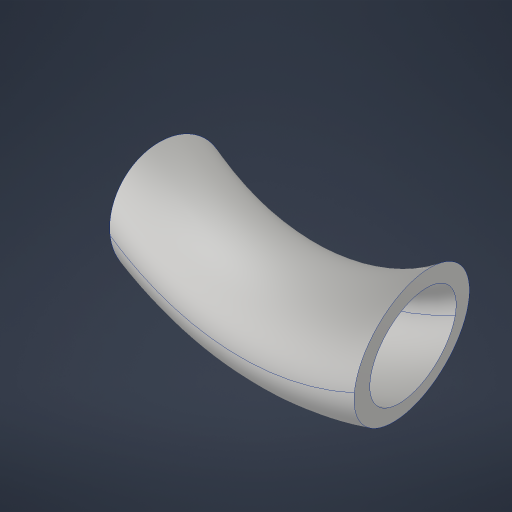
# Autodesk Inventor part: EL2-024
Saved by Autodesk Inventor 2023.4 (Build 274418000, 418)
## iProperties
Created: 2025-02-10
Part Number: EL2-024
Material: Aluminum 6061
Document SubType Name: Modeling
Designer: brand
Density: 2.7 g/cm^3
Appearance: Aluminum - Flat
Author: brand
Autodesk Inventor part; units mm, degrees
ref_plane "YZ Plane" through (0, 0, 0) normal (1, 0, 0) x (0, 1, 0)
ref_plane "XZ Plane" through (0, 0, 0) normal (0, 1, 0) x (-1, 0, 0)
ref_plane "XY Plane" through (0, 0, 0) normal (0, 0, 1) x (1, 0, 0)
sketch "Sketch1" plane through (0, 0, 0) normal (0, 0, 1) x (1, 0, 0)
  line L0 (-50.8, -41.275) -> (50.8, -41.275)
  line L1 (50.8, -41.275) -> (50.8, 41.275)
  line L2 (50.8, 41.275) -> (-50.8, 41.275)
  line L3 (-50.8, 41.275) -> (-50.8, -41.275)
  line L4 (-50.8, -41.275) -> (50.8, 41.275) construction
  line L5 (50.8, -41.275) -> (-50.8, 41.275) construction
  point P0 (0, 0)
  dimension "d0" = 101.6
  dimension "d1" = 82.55
  constraints: 12 end point, 2 midpoint, 2 parallel, 1 horizontal, 1 perpendicular
  measures "d0" distance of L2.end L1.end
  measures "d1" distance of L1.end L0.end
extrude "Extrusion1" add sketch "Sketch1" along normal mid plane 50.8
sketch "Sketch2" plane through (50.8, -41.275, 25.4) normal (1, 0, 0) x (0, 0, -1)
  line L0 (50.8, 82.55) -> (50.8, 0) construction
  line L1 (50.8, 0) -> (0, 0) construction
  line L2 (0, 0) -> (0, 82.55) construction
  line L3 (0, 82.55) -> (50.8, 82.55) construction
  circle A0 centre (25.4, 41.275) radius 19.05
  line L4 (50.8, 82.55) -> (0, 82.55) construction
  dimension "d4" = 38.1
  constraints: 3 coincident, 1 centre point
  measures "d4" diameter of A0
sketch "Sketch3" plane through (0, 0, 0) normal (0, 0, 1) x (1, 0, 0)
  line L0 (50.8, -41.275) -> (-50.8, -41.275) construction
  line L1 (-50.8, -41.275) -> (-50.8, 41.275) construction
  line L2 (-50.8, 41.275) -> (50.8, 41.275) construction
  line L3 (50.8, 41.275) -> (50.8, -41.275) construction
  arc A0 (-50.8, 0) -> (50.8, 0) centre (0, 80.5725) ccw construction
  circle A1 centre (0, 80.5725) radius 95.25
  point P0 (0, 0)
  dimension "d5" = 95.25
  constraints: 2 centre point, 2 point on circle, 1 coincident, 1 concentric, 1 horizontal alignment, 1 midpoint
  measures "d5" radius of A0
sweep "Sweep1" cut profiles "Sketch2" path "Sketch3"
sketch "Sketch7" plane through (50.8, -41.275, 25.4) normal (1, 0, 0) x (0, 0, -1)
  circle A0 centre (25.4, 41.275) radius 19.05 construction
  line L0 (50.8, 82.55) -> (50.8, 0) construction
  line L1 (50.8, 0) -> (0, 0) construction
  line L2 (0, 0) -> (0, 82.55) construction
  line L3 (0, 82.55) -> (50.8, 82.55) construction
  circle A1 centre (25.4, 41.275) radius 25.4
  line L4 (0, 0) -> (0, 82.55) construction
  line L5 (0, 41.275) -> (50.8, 41.275)
  line L6 (50.8, 41.275) -> (50.8, 107.95)
  line L7 (50.8, 107.95) -> (0, 107.95)
  line L8 (0, 107.95) -> (0, 41.275)
  line L9 (50.8, 82.55) -> (50.8, 0) construction
  line L10 (0, 41.275) -> (50.8, 41.275)
  line L11 (50.8, 41.275) -> (50.8, -25.4)
  line L12 (50.8, -25.4) -> (0, -25.4)
  line L13 (0, -25.4) -> (0, 41.275)
  point P0 (25.4, 41.275)
  point P1 (25.4, -25.4)
  dimension "d20" = 6.35
  dimension "d21" = 25.4
  dimension "d22" = 25.4
  constraints: 16 end point, 4 midpoint, 4 parallel, 2 horizontal, 2 perpendicular, 2 point on circle, 1 centre point, 1 coincident
  measures "d20" radial gap between concentric circles of A1 A0
  measures "d21" distance between parallel lines of L7 L3
  measures "d22" distance from line of point (25.4, -25.4) L1
sweep "Sweep5" cut profiles "Sketch7" path "Sketch3" contours A1 L8 L7 L6
sweep "Sweep6" cut profiles "Sketch7" path "Sketch3" contours L11 L12 L13 A1
sketch "Sketch8" plane through (0, 0, 25.4) normal (0, 0, 1) x (1, 0, 0)
  arc A0 (-35.0641, 41.275) -> (35.0641, 41.275) centre (0, 80.5725) ccw construction
  line L0 (-35.0641, 41.275) -> (35.0641, 41.275)
  line L1 (35.0641, 41.275) -> (35.0641, 27.9058)
  line L2 (35.0641, 27.9058) -> (-35.0641, 27.9058)
  line L3 (-35.0641, 27.9058) -> (-35.0641, 41.275)
  arc A1 (-50.8, 0) -> (50.8, 0) centre (0, 80.5725) ccw construction
  arc A2 (-35.0641, 41.275) -> (35.0641, 41.275) centre (0, 80.5725) ccw construction
  line L4 (-35.0641, 41.275) -> (35.0641, 41.275) construction
  arc A3 (-35.0641, 41.275) -> (35.0641, 41.275) centre (0, 80.5725) ccw construction
  point P0 (0, 0)
  constraints: 8 end point, 2 parallel, 1 horizontal, 1 perpendicular, 1 point on line, 1 tangent
extrude "Extrusion3" cut sketch "Sketch8" against normal through all
equation "\"d22\" = d21"
body "Solid1"
